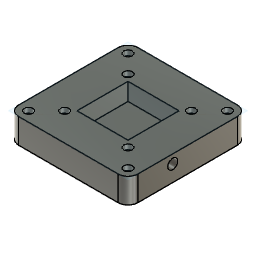
Fan_Base_New v6 (Autodesk Fusion 360 design; units mm, degrees)
Autodesk Fusion 360 part; units mm, degrees
note: some values were not read from the file. Set by a fixed rule: which sketch regions a step uses.
sketch "Sketch1" plane through (0, 0, 0) normal (0, 0, 1) x (1, 0, 0)
  line L0 (0, 0) -> (-48, 0)
  line L1 (-48, 0) -> (-48, 48)
  line L2 (-48, 48) -> (0, 48)
  line L3 (0, 48) -> (0, 0)
  dimension "d1" = 48
  dimension "d2" = 48
  constraint horizontal L0
  constraint vertical L1
  constraint horizontal L2
  constraint vertical L3
  constraint coincident L0.start L3.end
  measures "d1" distance of L0.start L0.end
  measures "d2" distance of L0.start L2.end
extrude "Extrude1" add sketch "Sketch1" along normal blind 10
sketch "Sketch2" plane through (0, 0, 10) normal (0, 0, 1) x (-1, 0, 0)
  line L0 (0, -48) -> (48, -48)
  line L1 (48, -48) -> (48, 0)
  line L2 (48, 0) -> (0, 0)
  line L3 (0, 0) -> (0, -48)
  line L4 (34.25, -13.75) -> (13.75, -13.75)
  line L5 (13.75, -13.75) -> (13.75, -34.25)
  line L6 (13.75, -34.25) -> (34.25, -34.25)
  line L7 (34.25, -34.25) -> (34.25, -13.75)
  line L8 (34.25, -13.75) -> (13.75, -34.25) construction
  line L9 (13.75, -13.75) -> (34.25, -34.25) construction
  point P0 (24, -24)
  dimension "d5" = 20.5
  dimension "d6" = 20.5
  constraint horizontal L4
  constraint perpendicular L4 L5
  constraint parallel L4 L6
  constraint parallel L5 L7
  constraint coincident L8 P0
  constraint coincident L9 P0
  measures "d5" distance of L5.end L6.end
  measures "d6" distance of L4.end L5.end
extrude "Extrude2" cut sketch "Sketch2" against normal blind 7 contours L4 L5 L6 L7
sketch "Sketch3" plane through (0, 0, 10) normal (0, 0, 1) x (-1, 0, 0)
  line L0 (13.75, -13.75) -> (34.25, -13.75)
  line L1 (34.25, -13.75) -> (34.25, -34.25)
  line L2 (34.25, -34.25) -> (13.75, -34.25)
  line L3 (13.75, -34.25) -> (13.75, -13.75)
  line L4 (0, -48) -> (48, -48)
  line L5 (48, -48) -> (48, 0)
  line L6 (48, 0) -> (0, 0)
  line L7 (0, 0) -> (0, -48)
sketch "Sketch4" plane through (0, 0, 0) normal (1, 0, 0) x (0, 1, 0)
  line L0 (0, 0) -> (48, 0)
  line L1 (48, 0) -> (48, 10)
  line L2 (48, 10) -> (0, 10)
  line L3 (0, 10) -> (0, 0)
  line L4 (0, 10) -> (18, 10)
  line L5 (18, 10) -> (18, 6.5)
  line L6 (18, 6.5) -> (0, 6.5)
  line L7 (0, 6.5) -> (0, 10)
  circle A0 centre (18, 6.5) radius 2
  dimension "d9" = 18
  dimension "d10" = 3.5
  dimension "d11" = 4
  constraint horizontal L4
  constraint vertical L5
  constraint horizontal L6
  constraint vertical L7
  constraint coincident L2.end L3.start
  constraint coincident L5.end L6.start
  measures "d9" distance of L2.end L4.end
  measures "d10" distance of L2.end L6.end
  measures "d11" diameter of A0
extrude "Extrude3" cut sketch "Sketch4" against normal blind 15 contours L5 L6 A0 | L5 L6 A0
fillet "Fillet1" radius 4 1 edges at (0, 48, 5)
fillet "Fillet2" radius 4 1 edges at (0, 0, 5)
fillet "Fillet3" radius 4 2 edges at (-48, 48, 5) (-48, 0, 5)
sketch "Sketch5" plane through (0, 0, 10) normal (0, 0, 1) x (-1, 0, 0)
  line L0 (13.75, -13.75) -> (11.25, -13.75)
  line L1 (11.25, -13.75) -> (11.25, -11.25)
  line L2 (11.25, -11.25) -> (13.75, -11.25)
  line L3 (13.75, -11.25) -> (13.75, -13.75)
  line L4 (11.25, -11.25) -> (36.75, -11.25)
  line L5 (36.75, -11.25) -> (36.75, -36.75)
  line L6 (36.75, -36.75) -> (11.25, -36.75)
  line L7 (11.25, -36.75) -> (11.25, -11.25)
  circle A0 centre (36.75, -36.75) radius 1.6
  circle A1 centre (11.25, -36.75) radius 1.6
  circle A2 centre (11.25, -11.25) radius 1.6
  circle A3 centre (36.75, -11.25) radius 1.6
  point P0 (13.75, -13.75)
  dimension "d20" = 2.5
  dimension "d21" = 2.5
  dimension "d22" = 25.5
  dimension "d23" = 25.5
  dimension "d24" = 3.2
  dimension "d25" = 3.2
  dimension "d26" = 3.2
  dimension "d27" = 3.2
  constraint horizontal L0
  constraint vertical L1
  constraint horizontal L2
  constraint vertical L3
  constraint coincident P0 L0.start
  constraint horizontal L4
  constraint vertical L5
  constraint horizontal L6
  constraint vertical L7
  constraint coincident L5.end L6.start
  constraint coincident L6.end L7.start
  constraint coincident L1.end L2.start
  constraint coincident L4.end L5.start
  measures "d20" distance of P0 L0.end
  measures "d21" distance of P0 L2.end
  measures "d22" distance of L1.end L4.end
  measures "d23" distance of L1.end L6.end
  measures "d24" diameter of A0
  measures "d25" diameter of A1
  measures "d26" diameter of A2
  measures "d27" diameter of A3
extrude "Extrude4" cut sketch "Sketch5" against normal blind 2 contours L1 L2 L4 L7 A2 | L1 L2 L4 L7 A2 | L6 L7 A1 | L6 L7 A1 | L4 L5 A3 | L4 L5 A3 | L5 L6 A0 | L5 L6 A0
sketch "Sketch6" plane through (0, 0, 0) normal (0, 0, -1) x (1, 0, 0)
  arc A0 (-44, 0) -> (-48, -4) centre (-44, -4) ccw
  line L0 (-48, -4) -> (-48, -44)
  arc A1 (-48, -44) -> (-44, -48) centre (-44, -44) ccw
  line L1 (-44, -48) -> (-4, -48)
  arc A2 (-4, -48) -> (0, -44) centre (-4, -44) ccw
  line L2 (0, -44) -> (0, -4)
  arc A3 (0, -4) -> (-4, 0) centre (-4, -4) ccw
  line L3 (-4, 0) -> (-44, 0)
  line L4 (0, 0) -> (-4, 0)
  line L5 (0, -4) -> (0, 0)
  circle A4 centre (-4, -44) radius 1.5
  circle A5 centre (-44, -44) radius 1.5
  circle A6 centre (-44, -4) radius 1.5
  circle A7 centre (-4, -4) radius 1.5
  dimension "d30" = 4
  dimension "d31" = 40
  dimension "d33" = 3
  dimension "d34" = 3
  dimension "d35" = 3
  dimension "d36" = 3
  constraint horizontal L4
  constraint vertical L5
  constraint coincident L4.start L5.end
  constraint concentric A2 A4
  constraint concentric A1 A5
  constraint concentric A3 A7
  measures "d30" distance of L4.start A3.end
  measures "d31" distance of A3.centre A0.centre
  measures "d33" diameter of A4
  measures "d34" diameter of A5
  measures "d35" diameter of A6
  measures "d36" diameter of A7
extrude "Extrude5" add sketch "Sketch6" along normal blind 2 contours A4 | A5 | A6 | A7
sketch "Sketch7" plane through (0, 0, 10) normal (0, 0, 1) x (-1, 0, 0)
  line L0 (0, 0) -> (4, 0)
  line L1 (4, 0) -> (4, -4)
  line L2 (4, -4) -> (0, -4)
  line L3 (0, -4) -> (0, 0)
  line L4 (4, -4) -> (44, -4)
  line L5 (44, -4) -> (44, -44)
  line L6 (44, -44) -> (4, -44)
  line L7 (4, -44) -> (4, -4)
  circle A0 centre (4, -4) radius 1.6
  circle A1 centre (44, -4) radius 1.6
  circle A2 centre (4, -44) radius 1.6
  circle A3 centre (44, -44) radius 1.6
  dimension "d39" = 4
  dimension "d40" = 4
  dimension "d41" = 40
  dimension "d42" = 40
  dimension "d43" = 3.2
  dimension "d44" = 3.2
  dimension "d45" = 3.2
  dimension "d46" = 3.2
  constraint horizontal L0
  constraint vertical L1
  constraint horizontal L2
  constraint vertical L3
  constraint coincident L0.start L3.end
  constraint horizontal L4
  constraint vertical L5
  constraint horizontal L6
  constraint vertical L7
  constraint coincident L1.end L2.start
  constraint coincident L4.end L5.start
  constraint coincident L6.end L7.start
  constraint coincident L5.end L6.start
  measures "d39" distance of L0.start L0.end
  measures "d40" distance of L0.start L2.end
  measures "d41" distance of L1.end L4.end
  measures "d42" distance of L1.end L6.end
  measures "d43" diameter of A0
  measures "d44" diameter of A1
  measures "d45" diameter of A2
  measures "d46" diameter of A3
extrude "Extrude6" cut sketch "Sketch7" against normal blind 2 contours L1 L4 A0 | L1 L2 A0 | L2 L7 A0 | L4 L7 A0 | L4 L5 A1 | L4 L5 A1 | L6 L7 A2 | L6 L7 A2 | L5 L6 A3 | L5 L6 A3
extrude "Extrude7" cut 4 faces at (-44.3721, 3.7344, -2) (-4.5584, 4.2485, -2) (-4.4413, 44.3401, -2) (-43.9601, 44.4654, -2) along direction (0, 0, 1) blind 2
sketch "Sketch8" plane through (0, 0, 0) normal (0, 0, -1) x (1, 0, 0)
  arc A0 (-44, 0) -> (-48, -4) centre (-44, -4) ccw
  line L0 (-48, -4) -> (-48, -44)
  arc A1 (-48, -44) -> (-44, -48) centre (-44, -44) ccw
  line L1 (-44, -48) -> (-4, -48)
  arc A2 (-4, -48) -> (0, -44) centre (-4, -44) ccw
  line L2 (0, -44) -> (0, -4)
  arc A3 (0, -4) -> (-4, 0) centre (-4, -4) ccw
  line L3 (-4, 0) -> (-44, 0)
  line L4 (0, 0) -> (-4, 0)
  line L5 (-4, 0) -> (-4, -4)
  line L6 (-4, -4) -> (0, -4)
  line L7 (0, -4) -> (0, 0)
  line L8 (-4, -4) -> (-44, -4)
  line L9 (-44, -4) -> (-44, -44)
  line L10 (-44, -44) -> (-4, -44)
  line L11 (-4, -44) -> (-4, -4)
  circle A4 centre (-24, -4) radius 1.5
  circle A5 centre (-24, -44) radius 1.5
  circle A6 centre (-4, -24) radius 1.5
  circle A7 centre (-44, -24) radius 1.5
  dimension "d51" = 4
  dimension "d52" = 40
  dimension "d53" = 40
  dimension "d54" = 3
  dimension "d55" = 3
  dimension "d56" = 3
  dimension "d57" = 3
  constraint horizontal L4
  constraint vertical L5
  constraint horizontal L6
  constraint vertical L7
  constraint coincident L4.start L7.end
  constraint horizontal L8
  constraint vertical L9
  constraint horizontal L10
  constraint vertical L11
  constraint coincident A3.centre L5.end
  constraint midpoint L8 A4.centre
  constraint midpoint L10 A5.centre
  constraint midpoint L11 A6.centre
  constraint midpoint L9 A7.centre
  measures "d51" distance of L4.start A3.end
  measures "d52" distance of A3.centre A0.centre
  measures "d53" distance of A3.centre A2.centre
  measures "d54" diameter of A4
  measures "d55" diameter of A5
  measures "d56" diameter of A6
  measures "d57" diameter of A7
extrude "Extrude8" add sketch "Sketch8" along normal blind 2 contours L8 A4 | L8 A4 | L11 A6 | L11 A6 | L9 A7 | L9 A7 | L10 A5 | L10 A5
sketch "Sketch9" plane through (0, 0, 10) normal (0, 0, 1) x (-1, 0, 0)
  circle A0 centre (4, -4) radius 1.7
  dimension "d60" = 3.4
  measures "d60" diameter of A0
extrude "Extrude9" cut sketch "Sketch9" against normal blind 2
sketch "Sketch10" plane through (0, 0, 10) normal (0, 0, 1) x (-1, 0, 0)
  circle A0 centre (4, -44) radius 1.7
  arc A1 (0, -44) -> (4, -48) centre (4, -44) ccw
  dimension "d63" = 3.4
  constraint concentric A0 A1
  measures "d63" diameter of A0
extrude "Extrude10" cut sketch "Sketch10" against normal blind 2
sketch "Sketch11" plane through (0, 0, 10) normal (0, 0, 1) x (-1, 0, 0)
  circle A0 centre (44, -4) radius 1.7
  dimension "d66" = 3.4
  measures "d66" diameter of A0
extrude "Extrude11" cut sketch "Sketch11" against normal blind 2
sketch "Sketch12" plane through (0, 0, 10) normal (0, 0, 1) x (-1, 0, 0)
  circle A0 centre (44, -44) radius 1.7
  dimension "d69" = 3.4
  measures "d69" diameter of A0
extrude "Extrude12" cut sketch "Sketch12" against normal blind 2
sketch "Sketch13" plane through (0, 0, 10) normal (0, 0, 1) x (-1, 0, 0)
  circle A0 centre (11.25, -11.25) radius 1.7
  circle A1 centre (11.25, -11.25) radius 1.6
  dimension "d72" = 3.4
  constraint concentric A0 A1
  measures "d72" diameter of A0
extrude "Extrude13" cut sketch "Sketch13" against normal blind 2
sketch "Sketch14" plane through (0, 0, 10) normal (0, 0, 1) x (-1, 0, 0)
  circle A0 centre (36.75, -11.25) radius 1.7
  circle A1 centre (36.75, -11.25) radius 1.6
  dimension "d75" = 3.4
  constraint concentric A0 A1
  measures "d75" diameter of A0
extrude "Extrude14" cut sketch "Sketch14" against normal blind 2
sketch "Sketch15" plane through (0, 0, 10) normal (0, 0, 1) x (-1, 0, 0)
  circle A0 centre (36.75, -36.75) radius 1.7
  circle A1 centre (36.75, -36.75) radius 1.6
  dimension "d78" = 3.4
  constraint concentric A0 A1
  measures "d78" diameter of A0
extrude "Extrude15" cut sketch "Sketch15" against normal blind 2
sketch "Sketch16" plane through (0, 0, 10) normal (0, 0, 1) x (-1, 0, 0)
  circle A0 centre (11.25, -36.75) radius 1.7
  circle A1 centre (11.25, -36.75) radius 1.6
  dimension "d81" = 3.4
  constraint concentric A0 A1
  measures "d81" diameter of A0
extrude "Extrude16" cut sketch "Sketch16" against normal blind 2
